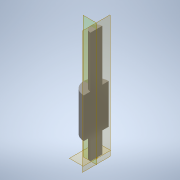
# Autodesk Inventor part: Stang
Saved by Autodesk Inventor 2021 (Build 250183000, 183)
## iProperties
Manager: PJ / DCS
Company: Emmaüs Bovenbouw Aalter
Created: 2021-01-10
Part Number: Stang
Material: S235
Catalog Web Link: http://emmausbovenbouw.op-weg.be/
Vendor: Emmaüsinstituut Bovenbouw Aalter
Document SubType Name: Modeling
Designer: Antho
Engineer: Declercq St.
Manufacturer: Standard
Standards Organization: Custom
Density: 7.86 g/cm^3
Appearance: Steel
Title: Algemene titel
Subject: Specifieke titel
Author: Antho
Keywords: Ruwe Ø xxxxx
Comments: Opmerking
Autodesk Inventor part; units mm, degrees
sketch "Sketch1" plane through (0, 0, 0) normal (0, 0, 1) x (1, 0, 0)
  line L0 (0, 2.0365) -> (0, -2.0365) construction
  line L1 (-4.1164, 0) -> (4.1164, 0) construction
  circle A0 centre (0, 0) radius 2.85
  dimension "d0" = 5.7
  constraints: 4 end point, 2 coincident, 2 midpoint, 1 centre point, 1 horizontal, 1 vertical
  measures "d0" diameter of A0
extrude "Extrusion1" add sketch "Sketch1" along normal blind 10
sketch "Sketch2" plane through (0, 0, 10) normal (0, 0, 1) x (1, 0, 0)
  circle A0 centre (0, 0) radius 6
  dimension "d3" = 12
  constraints: 1 centre point, 1 coincident
  measures "d3" diameter of A0
extrude "Extrusion2" add sketch "Sketch2" along normal blind 19
sketch "Sketch3" plane through (0, 0, 29) normal (0, 0, 1) x (1, 0, 0)
  circle A0 centre (0, 0) radius 2.85
  dimension "d6" = 5.7
  constraints: 1 centre point, 1 coincident
  measures "d6" diameter of A0
extrude "Extrusion3" add sketch "Sketch3" along normal blind 24.5
sketch "Sketch5" plane through (0, 0, 53.5) normal (0, 0, 1) x (1, 0, 0)
  line L0 (0, 8.3226) -> (8.1221, 8.3226)
  line L1 (8.1221, 8.3226) -> (8.1221, -8.0744)
  line L2 (8.1221, -8.0744) -> (0, -8.0744)
  line L3 (0, -8.0744) -> (0, 8.3226)
  point P0 (0, 0)
  constraints: 8 end point, 2 parallel, 1 horizontal, 1 perpendicular
extrude "Extrusion5" cut sketch "Sketch5" against normal blind 58
body "Solid1"
